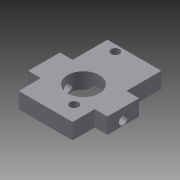
# Autodesk Inventor part: tapa0.2
Saved by Autodesk Inventor 2015 SP1 (Build 190203100, 203)
## iProperties
Created: 2015-06-09
Part Number: tapa0.2
Material: Generic
Document SubType Name: Modeling
Designer: pc
Density: 1 g/cm^3
Appearance: Default
Author: pc
Autodesk Inventor part; units mm, degrees
ref_plane "YZ Plane" through (0, 0, 0) normal (1, 0, 0) x (0, 1, 0)
ref_plane "XZ Plane" through (0, 0, 0) normal (0, 1, 0) x (-1, 0, 0)
ref_plane "XY Plane" through (0, 0, 0) normal (0, 0, 1) x (1, 0, 0)
sketch "Sketch2" plane through (0, 0, 0) normal (0, 0, 1) x (1, 0, 0)
  line L0 (-17, 28) -> (0, 28)
  line L1 (0, 28) -> (0, 17)
  line L2 (0, 17) -> (4, 17)
  line L3 (4, 17) -> (4, 7)
  line L4 (4, 7) -> (0, 7)
  line L5 (0, 7) -> (0, 0)
  line L6 (0, 0) -> (-17, 0)
  line L7 (-17, 0) -> (-17, 7)
  line L8 (-17, 7) -> (-21, 7)
  line L9 (-21, 7) -> (-21, 17)
  line L10 (-21, 17) -> (-17, 17)
  line L11 (-17, 28) -> (-17, 17)
  dimension "d0" = 17
  dimension "d1" = 28
  dimension "d2" = 4
  dimension "d3" = 7
  dimension "d4" = 10
  constraints: 24 end point, 7 point on line, 6 perpendicular, 3 horizontal, 1 coincident, 1 collinear
  measures "d0" distance of L0.start L0.end
  measures "d1" distance between parallel lines of L0 L6
  measures "d2" distance of L9.end L10.end
  measures "d3" distance of L6.end L7.end
  measures "d4" distance of L8.end L9.end
extrude "Extrusion1" add sketch "Sketch2" along normal blind 5
sketch "Sketch4" plane through (0, 0, 0) normal (0, 0, -1) x (-1, 0, 0)
  line L0 (17, 28) -> (0, 28) projected
  line L1 (0, 28) -> (0, 17) projected
  line L2 (0, 17) -> (-4, 17) projected
  line L3 (-4, 17) -> (-4, 7) projected
  line L4 (-4, 7) -> (0, 7) projected
  line L5 (0, 7) -> (0, 0) projected
  line L6 (0, 0) -> (17, 0) projected
  line L7 (17, 0) -> (17, 7) projected
  line L8 (17, 7) -> (21, 7) projected
  line L9 (21, 7) -> (21, 17) projected
  line L10 (21, 17) -> (17, 17) projected
  line L11 (17, 17) -> (17, 28) projected
  line L12 (0, 28) -> (17, 28) projected
  line L13 (11.5, 24) -> (11.5, 4)
  line L14 (11.5, 4) -> (5.5, 4)
  line L15 (5.5, 4) -> (5.5, 24)
  line L16 (5.5, 24) -> (11.5, 24)
  dimension "d15" = 6
  dimension "d17" = 5.5
  dimension "d30" = 20
  dimension "d31" = 4
  constraints: 8 end point, 1 parallel, 1 perpendicular
  measures "d15" distance of L13.end L14.end
  measures "d17" distance between parallel lines of L15 L1
  measures "d30" distance of L13.start L13.end
  measures "d31" distance between parallel lines of L6 L14
extrude "Extrusion3" cut sketch "Sketch4" against normal blind 1.5 contours L13 L14 L15 L16
sketch "Sketch5" plane through (0, 0, 5) normal (0, 0, 1) x (1, 0, 0)
  line L0 (0, 28) -> (-17, 28) projected
  line L1 (-17, 28) -> (-17, 17) projected
  line L2 (-17, 17) -> (-21, 17) projected
  line L3 (-21, 17) -> (-21, 7) projected
  line L4 (-21, 7) -> (-17, 7) projected
  line L5 (-17, 7) -> (-17, 0) projected
  line L6 (-17, 0) -> (0, 0) projected
  line L7 (0, 0) -> (0, 7) projected
  line L8 (0, 7) -> (4, 7) projected
  line L9 (4, 7) -> (4, 17) projected
  line L10 (4, 17) -> (0, 17) projected
  line L11 (0, 17) -> (0, 28) projected
  line L12 (-21, 17) -> (4, 7)
  line L13 (-21.4753, 7) -> (4, 17)
  circle A0 centre (-8.6177, 12.0471) radius 5
  dimension "d20" = 10
  dimension "d21" = 12.0471
  constraints: 4 end point, 2 point on line, 1 centre point
  measures "d20" diameter of A0
  measures "d21" distance from line of L6 A0.centre
extrude "Extrusion4" cut sketch "Sketch5" against normal through all contours A0 L12 L13 | L13 L12 A0 | L12 L13 A0 | A0 L13 L12
sketch "Sketch6" plane through (0, 0, 5) normal (0, 0, 1) x (1, 0, 0)
  circle A0 centre (-8.6177, 12.0471) radius 5 projected
  line L0 (0, 28) -> (-17, 28) projected
  line L1 (-17, 28) -> (-17, 17) projected
  line L2 (-17, 17) -> (-21, 17) projected
  line L3 (-21, 17) -> (-21, 7) projected
  line L4 (-21, 7) -> (-17, 7) projected
  line L5 (-17, 7) -> (-17, 0) projected
  line L6 (-17, 0) -> (0, 0) projected
  line L7 (0, 0) -> (0, 7) projected
  line L8 (0, 7) -> (4, 7) projected
  line L9 (4, 7) -> (4, 17) projected
  line L10 (4, 17) -> (0, 17) projected
  line L11 (0, 17) -> (0, 28) projected
  circle A1 centre (-12.5, 26) radius 1.35
  dimension "d24" = 2.7
  dimension "d25" = 4.5
  dimension "d26" = 2
  constraints: 1 centre point
  measures "d24" diameter of A1
  measures "d25" distance from line of A1.centre L1
  measures "d26" distance from line of L0 A1.centre
extrude "Extrusion5" cut sketch "Sketch6" against normal through all contours A1
sketch "Sketch7" plane through (0, 0, 5) normal (0, 0, 1) x (1, 0, 0)
  line L0 (0, 0) -> (0, 7) projected
  line L1 (-17, 0) -> (0, 0) projected
  circle A0 centre (-4.5, 5) radius 1.35
  dimension "d32" = 2.7
  dimension "d33" = 4.5
  dimension "d34" = 5
  constraints: 1 centre point
  measures "d32" diameter of A0
  measures "d33" distance from line of L0 A0.centre
  measures "d34" distance from line of L1 A0.centre
extrude "Extrusion6" cut sketch "Sketch7" against normal through all
sketch "Sketch8" plane through (4, 7, 0) normal (1, 0, 0) x (0, 0, -1)
  line L0 (0, 10) -> (0, 0) projected
  line L1 (0, 10) -> (-5, 10) projected
  line L2 (-5, 0) -> (-5, 10) projected
  line L3 (0, 0) -> (-5, 0) projected
  circle A0 centre (-1.5, 5) radius 1.35
  point P0 (0, -7)
  dimension "d37" = 2.7
  dimension "d38" = 1.5
  constraints: 1 centre point
  measures "d37" diameter of A0
  measures "d38" distance from line of L0 A0.centre
extrude "Extrusion7" cut sketch "Sketch8" against normal through all contours A0
body "Solid1"
